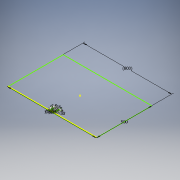
# Autodesk Inventor part: regla_digital
Saved by Autodesk Inventor 2018 (Build 220112000, 112)
## iProperties
Created: 2019-02-11
Part Number: regla_digital
Material: Generic
Document SubType Name: Modeling
Designer: zoticus
Density: 1 g/cm^3
Appearance: Default
Author: zoticus
Autodesk Inventor part; units mm, degrees
ref_plane "YZ Plane" through (0, 0, 0) normal (1, 0, 0) x (0, 1, 0)
ref_plane "XZ Plane" through (0, 0, 0) normal (0, 1, 0) x (-1, 0, 0)
ref_plane "XY Plane" through (0, 0, 0) normal (0, 0, 1) x (1, 0, 0)
sketch "Sketch1" plane through (0, 0, 0) normal (0, 0, 1) x (1, 0, 0)
  line L0 (-401.966, 248.4646) -> (398.034, 248.4646)
  line L1 (398.034, 248.4646) -> (398.034, -251.5354)
  line L2 (398.034, -251.5354) -> (-401.966, -251.5354)
  line L3 (-401.966, -251.5354) -> (-401.966, 248.4646)
  dimension "d0" = 800
  dimension "d1" = 500
  dimension "d2" = 800
  constraints: 8 end point, 2 parallel, 1 horizontal, 1 perpendicular
  measures "d0" distance of L1.end L2.end
  measures "d1" distance of L0.end L1.end
  measures "d2" distance of L0.end L0.start
extrude "Extrusion1" add sketch "Sketch1" along normal blind 5
sketch "Sketch2" plane through (0, 0, 5) normal (0, 0, 1) x (1, 0, 0)
  point P0 (0, 0)
sketch "Sketch3" plane through (0, 0, 5) normal (0, 0, 1) x (1, 0, 0)
  line L0 (-401.966, -251.5354) -> (398.034, -251.5354) projected
  point P0 (0, 0)
sketch "Sketch4" plane through (0, 0, 5) normal (0, 0, 1) x (1, 0, 0)
  line L0 (-401.966, -251.5354) -> (398.034, -251.5354) projected
  line L1 (-1.966, -251.5354) -> (-1.966, -241.0354)
  line L2 (-1.966, -241.0354) -> (6.534, -241.0354)
  line L3 (-1.966, -241.0354) -> (-10.466, -241.0354)
  point P0 (0, 0)
  dimension "d7" = 10.5
  dimension "d8" = 8.5
  dimension "d9" = 8.5
  constraints: 6 end point, 2 coincident, 1 horizontal, 1 midpoint, 1 perpendicular, 1 vertical
  measures "d7" distance of L1.start L1.end
  measures "d8" distance of L1.end L2.end
  measures "d9" distance of L1.end L3.end
hole "Hole1" at (6.534, -241.0354, 5) at (-10.466, -241.0354, 5) direction (0, 0, -1) diameter 3 depth 5 tip angle 118 counterbore diameter 6 counterbore depth 2.5
sketch "Sketch5" plane through (0, 0, 5) normal (0, 0, 1) x (1, 0, 0)
  point P0 (0, 0)
sketch "Sketch6" plane through (0, 0, 5) normal (0, 0, 1) x (1, 0, 0)
  line L0 (398.034, -251.5354) -> (-401.966, -251.5354) projected
  line L1 (6.5526, -251.5354) -> (6.5526, -248.0354)
  line L2 (0, -251.5354) -> (3.5, -251.5354) construction
  line L3 (-4.8949, -248.0354) -> (13.1051, -248.0354)
  line L4 (-4.8949, -248.0354) -> (-22.8949, -248.0354)
  line L5 (13.1051, -248.0354) -> (13.1051, -234.0354)
  circle A0 centre (-10.466, -241.0354) radius 1.5 projected
  line L6 (-10.466, -241.0354) -> (-16.966, -241.0354)
  line L7 (6.5526, -241.0354) -> (13.0526, -241.0354)
  line L8 (-22.8949, -248.0354) -> (-20.3949, -248.0354)
  line L9 (-20.3949, -248.0354) -> (-20.3949, -218.0354)
  line L10 (-20.3949, -218.0354) -> (-22.8949, -218.0354)
  line L11 (-22.8949, -218.0354) -> (-22.8949, -248.0354)
  line L12 (-22.8949, -248.0354) -> (-25.3949, -248.0354)
  line L13 (-25.3949, -248.0354) -> (-25.3949, -218.0354)
  line L14 (-25.3949, -218.0354) -> (-22.8949, -218.0354)
  line L15 (-22.8949, -218.0354) -> (-22.8949, -248.0354)
  line L16 (13.1051, -234.0354) -> (15.6051, -234.0354)
  line L17 (15.6051, -234.0354) -> (15.6051, -204.0354)
  line L18 (15.6051, -204.0354) -> (13.1051, -204.0354)
  line L19 (13.1051, -204.0354) -> (13.1051, -234.0354)
  line L20 (13.1051, -234.0354) -> (10.6051, -234.0354)
  line L21 (10.6051, -234.0354) -> (10.6051, -204.0354)
  line L22 (10.6051, -204.0354) -> (13.1051, -204.0354)
  line L23 (13.1051, -204.0354) -> (13.1051, -234.0354)
  point P0 (0, 0)
  dimension "d17" = 3.5
  dimension "d18" = 90
  dimension "d19" = 18
  dimension "d20" = 18
  dimension "d21" = 14
  dimension "d22" = 6.5
  dimension "d23" = 6.5
  dimension "d24" = 2.5
  dimension "d25" = 30
  dimension "d26" = 2.5
  dimension "d27" = 2.5
  dimension "d28" = 30
  dimension "d29" = 2.5
  dimension "d30" = 30
  dimension "d52" = 36
  dimension "d53" = 17.0186
  constraints: 46 end point, 8 parallel, 7 horizontal, 7 perpendicular, 4 coincident, 2 point on line, 1 vertical
  measures "d17" distance of L1.end L1.start
  measures "d18" angle of L2 L1
  measures "d19" distance of L3.start L3.end
  measures "d20" distance of L3.start L4.end
  measures "d21" distance of L5.start L5.end
  measures "d22" distance of L6.start L6.end
  measures "d23" distance of L7.start L7.end
  measures "d24" distance of L10.end L9.end
  measures "d25" distance of L9.end L8.end
  measures "d26" distance of L13.end L14.end
  measures "d27" distance of L18.end L17.end
  measures "d28" distance of L17.end L16.end
  measures "d29" distance of L21.end L22.end
  measures "d30" distance of L20.end L21.end
  measures "d52" horizontal distance of L18.end L10.end
  measures "d53" distance of L7.start L6.start
sketch "Sketch7" plane through (0, 0, 0) normal (0, 0, -1) x (-1, 0, 0)
  point P0 (0, 0)
hole "Hole2" at (-22.8949, -248.0354, 5) at (13.1051, -234.0354, 5) direction (0, 0, -1) diameter 5 depth 15 tip angle 118
extrude "Extrusion2" cut sketch "Sketch6" against normal blind 15 contours L20 L21 L22 L19 | L19 L18 L17 L16 | L4 L11 L10 L9 | L12 L13 L14 L11
hole "Hole3" at (-22.8949, -218.0354, 5) at (13.1051, -204.0354, 5) direction (0, 0, -1) diameter 5 depth 15 tip angle 118
sketch "Sketch8" plane through (0, 0, 5) normal (0, 0, 1) x (1, 0, 0)
  line L0 (398.034, -251.5354) -> (-401.966, -251.5354) projected
  line L1 (-45.2231, -251.5354) -> (34.7769, -251.5354)
  line L2 (34.7769, -251.5354) -> (34.7769, -191.5354)
  line L3 (34.7769, -191.5354) -> (-45.2231, -191.5354)
  line L4 (-45.2231, -191.5354) -> (-45.2231, -251.5354)
  line L5 (-45.2231, 276.0506) -> (-471.5877, 276.0506)
  line L6 (-471.5877, 276.0506) -> (-471.5877, -297.567)
  line L7 (-471.5877, -297.567) -> (-45.2231, -297.567)
  line L8 (-45.2231, -297.567) -> (-45.2231, 276.0506)
  line L9 (-45.2231, -191.5354) -> (471.8148, -191.5354)
  line L10 (471.8148, -191.5354) -> (471.8148, 308.5195)
  line L11 (471.8148, 308.5195) -> (-45.2231, 308.5195)
  line L12 (-45.2231, 308.5195) -> (-45.2231, -191.5354)
  line L13 (34.7769, -191.5354) -> (471.8148, -191.5354)
  line L14 (471.8148, -191.5354) -> (471.8148, -324.6244)
  line L15 (471.8148, -324.6244) -> (34.7769, -324.6244)
  line L16 (34.7769, -324.6244) -> (34.7769, -191.5354)
  point P0 (0, 0)
  dimension "d48" = 80
  dimension "d49" = 60
  constraints: 32 end point, 8 parallel, 4 horizontal, 4 perpendicular, 3 point on line
  measures "d48" distance of L3.end L2.end
  measures "d49" distance of L2.end L1.end
extrude "Extrusion3" cut sketch "Sketch8" against normal blind 15 contours L2 L9 L14 L15 L16 | L8 L7 L6 L5 L4 | L3 L8 L12 L11 L10 L9
body "Solid1"
